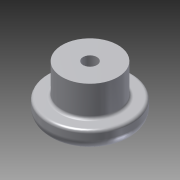
# Autodesk Inventor part: pied
Saved by Autodesk Inventor 2014 SP2 (Build 180246200, 246)
## iProperties
Created: 2015-03-18
Part Number: pied
Material: Plastique ABS
Document SubType Name: Modeling
Designer: sd
Density: 1.06 g/cm^3
Appearance: Lisse - Blanc
Mass: 0.630083 g
Surface Area: 5.06401 cm^2
Volume: 0.594418 cm^3
Author: sd
Autodesk Inventor part; units mm, degrees
ref_plane "YZ Plane" through (0, 0, 0) normal (1, 0, 0) x (0, 1, 0)
ref_plane "XZ Plane" through (0, 0, 0) normal (0, 1, 0) x (-1, 0, 0)
ref_plane "XY Plane" through (0, 0, 0) normal (0, 0, 1) x (1, 0, 0)
sketch "Esquisse1" plane through (0, 0, 0) normal (0, 1, 0) x (-1, 0, 0)
  line L0 (0, -6.7291) -> (0, 2.2709)
  line L1 (0, 2.2709) -> (-5, 2.2709)
  line L2 (-5, 2.2709) -> (-5, -3.2291)
  line L3 (-5, -3.2291) -> (-7.5, -3.2291)
  line L4 (0, -6.7291) -> (-7.5, -6.7291)
  line L5 (-7.5, -3.2291) -> (-7.5, -6.7291)
  point P0 (0, 0)
  dimension "d0" = 9
  dimension "d1" = 5
  dimension "d2" = 5.5
  dimension "d3" = 7.5
  constraints: 12 end point, 3 parallel, 2 perpendicular, 1 vertical
  measures "d0" distance of L0.start L0.end
  measures "d1" distance of L0.end L1.end
  measures "d2" distance of L1.end L2.end
  measures "d3" distance of L0.start L4.end
revolve "Révolution1" add sketch "Esquisse1" angle 360 about axis through (0, 0, -6.7291) along (0, 0, 1)
fillet "Congé1" radius 2 1 edges at (-7.5, 0, -6.7291)
fillet "Congé2" radius 0.5 1 edges at (-7.5, 0, -3.2291)
fillet "Congé3" radius 0.5 1 edges at (-5, 0, -3.2291)
hole "Perçage1" at (0, 0, 2.2709) direction (0, 0, -1) diameter 2.5 depth 7
